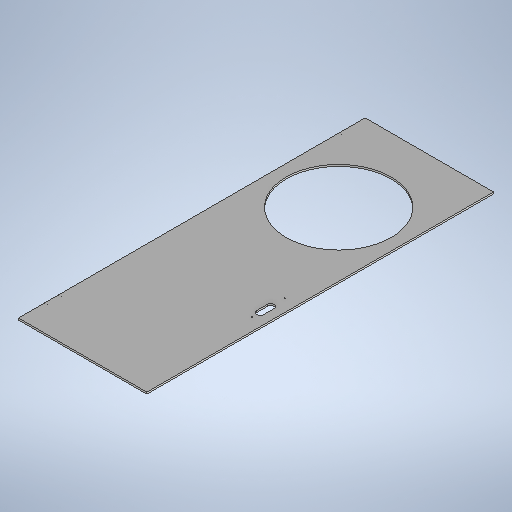
# Autodesk Inventor part: Rahmen
Saved by Autodesk Inventor 2025.1 (Build 291241000, 241)
## iProperties
Created: 2024-08-07
Part Number: Rahmen
Material: Generic
Document SubType Name: Modeling
Designer: ffogue
Density: 1 g/cm^3
Appearance: Default
Author: ffogue
Autodesk Inventor part; units mm, degrees
ref_plane "YZ Plane" through (0, 0, 0) normal (1, 0, 0) x (0, 1, 0)
ref_plane "XY Plane" through (0, 0, 0) normal (0, 0, 1) x (1, 0, 0)
sketch "Sketch4" plane through (0, 0, 0) normal (0, 0, 1) x (1, 0, 0)
  line L0 (0, 0) -> (735, 0)
  line L1 (735, 0) -> (735, 1985)
  line L2 (735, 1985) -> (0, 1985)
  line L3 (0, 1985) -> (0, 0)
  dimension "d0" = 735
  dimension "d1" = 1985
  constraints: 8 end point, 2 parallel, 1 coincident, 1 perpendicular
  measures "d0" distance between parallel lines of L1 L3
  measures "d1" distance between parallel lines of L0 L2
extrude "Extrusion1" add sketch "Sketch4" along normal blind 10
sketch "Sketch5" plane through (0, 0, 10) normal (0, 0, 1) x (1, 0, 0)
  circle A0 centre (367.5, 1466) radius 300
  line L0 (735, 1985) -> (0, 1985) projected
  point P0 (0, 0)
  point P1 (367.5, 1985)
  dimension "d4" = 600
  dimension "d5" = 519
  constraints: 1 centre point, 1 midpoint, 1 vertical alignment
  measures "d4" diameter of A0
  measures "d5" distance from line of A0.centre L0
extrude "Extrusion2" cut sketch "Sketch5" against normal up to surface (10 mm away)
sketch "Sketch6" plane through (0, 0, 0) normal (0, 0, -1) x (-1, 0, 0)
  line L0 (-665, 720) -> (-665, 780) construction
  line L1 (-645, 720) -> (-645, 780)
  line L2 (-685, 780) -> (-685, 720)
  arc A0 (-685, 720) -> (-645, 720) centre (-665, 720) ccw
  arc A1 (-645, 780) -> (-685, 780) centre (-665, 780) ccw
  line L3 (0, 0) -> (-735, 0) projected
  line L4 (-735, 0) -> (-735, 1985) projected
  circle A2 centre (-665, 860) radius 3.5
  circle A3 centre (-665, 673) radius 3.5
  point P0 (-665, 750)
  point P1 (-665, 700)
  point P2 (-665, 800)
  dimension "d8" = 700
  dimension "d9" = 50
  dimension "d10" = 40
  dimension "d11" = 100
  dimension "d12" = 7
  dimension "d13" = 60
  dimension "d16" = 187
  dimension "d17" = 7
  constraints: 8 end point, 6 point on circle, 4 centre point, 4 tangent, 2 vertical alignment, 1 midpoint, 1 parallel, 1 vertical
  measures "d8" distance from line of L3 point (-665, 700)
  measures "d9" distance between parallel lines of L4 L2
  measures "d10" distance between parallel lines of L1 L2
  measures "d11" distance of point (-665, 700) point (-665, 800)
  measures "d12" diameter of A2
  measures "d13" distance of A2.centre point (-665, 800)
  measures "d16" distance of A3.centre A2.centre
  measures "d17" diameter of A3
extrude "Extrusion3" cut sketch "Sketch6" against normal blind 10 contours A0 L2 A1 L1 | A2
extrude "Extrusion4" cut sketch "Sketch6" against normal up to surface (10 mm away) contours A3
sketch "Sketch7" plane through (0, 0, 0) normal (-1, 0, 0) x (0, 0, 1)
  circle A0 centre (5, 150) radius 3
  circle A1 centre (5, 230) radius 3
  line L0 (0, 0) -> (10, 0) projected
  point P0 (5, 0)
  dimension "d21" = 150
  dimension "d22" = 80
  dimension "d23" = 6
  constraints: 2 centre point, 2 vertical alignment, 1 equal radius, 1 midpoint
  measures "d21" distance from line of L0 A0.centre
  measures "d22" distance of A0.centre A1.centre
  measures "d23" diameter of A1
extrude "Extrusion5" cut sketch "Sketch7" against normal blind 15
thread "Thread1" size "M6x1" class "6H" standard "ISO Metric profile" length 10
thread "Thread2" size "M6x1" class "6H" standard "ISO Metric profile" length 10
ref_plane "Work Plane1" through (0, 992.5, 0) normal (0, 1, 0) x (-1, 0, 0)
mirror "Mirror1" about plane through (0, 992.5, 0) normal (0, 1, 0) of "Extrusion5"
equation "\"d0\" = RahmBrei"
equation "\"d1\" = RahmHoeh"
equation "\"d2\" = RahmDick"
equation "\"RahmBrei\" = 735"
equation "\"RahmHoeh\" = 1985"
equation "\"RahmDick\" = 10"
body "Solid1"
